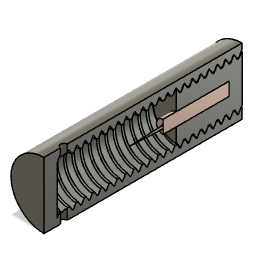
gasChargingBombHolderSchnittbild v2 (Autodesk Fusion 360 design; units mm, degrees)
Autodesk Fusion 360 part; units mm, degrees
sketch "Skizze1" plane through (0, 0, 0) normal (0, 0, 1) x (1, 0, 0)
  circle A0 centre (0, 0) radius 5
  dimension "d1" = 10
  constraint coincident A0.centre origin
  measures "d1" diameter of A0
extrude "Extrusion1" add sketch "Skizze1" along normal blind 10 makes body 1
sketch "Skizze8" plane through (0, 0, 10) normal (0, 0, 1) x (1, 0, 0)
  circle A0 centre (0, 0) radius 5
  circle A1 centre (0, 0) radius 1
  dimension "d45" = 2
  constraint coincident A0.centre A1.centre
  measures "d45" diameter of A1
extrude "Extrusion6" cut sketch "Skizze8" against normal blind 8 contours A1 bodies 1
thread "Gewinde5" "ISO Metric profile 8.0 M8x1.25 6g" major diameter 7.866 minor diameter 6.4455 pitch 1.25 angle 60 modelled right hand crest width 0.1833 on face at (4.9938, -0.2492, 6.6667) crest through (3.933, 0, -0.3125) on bodies 1
sketch "Skizze1 (2)" plane through (0, 0, 0) normal (0, 0, 1) x (1, 0, 0) in component "gasChargingBombLid v4"
  circle A0 centre (0, 0) radius 5
  dimension "d1_1" = 10
  constraint coincident A0.centre origin
  measures "d1_1" diameter of A0
extrude "Extrusion1'" add sketch "Skizze1 (2)" along normal blind 30 separate body makes body 2 in component "gasChargingBombLid v4"
ref_plane "Arbeitsebene1" through (0, 5, 2.1001) normal (0, 1, 0) x (1, 0, 0) in component "gasChargingBombLid v4"
sketch "Skizze3" plane through (0, 5, 2.1001) normal (0, 1, 0) x (1, 0, 0) in component "gasChargingBombLid v4"
  line L0 (-5, 2.1001) -> (5, 2.1001)
  circle A0 centre (0, -0.8999) radius 0.5
  dimension "d16" = 1
  dimension "d17" = 3
  measures "d16" diameter of A0
  measures "d17" distance of L0 A0.centre
sketch "Skizze4" plane through (0, 0, 30) normal (0, 0, 1) x (1, 0, 0) in component "gasChargingBombLid v4"
  circle A0 centre (0, 0) radius 5
  circle A1 centre (0, 0) radius 3.9
  dimension "d12" = 7.8
  constraint concentric A0 A1
  measures "d12" diameter of A1
extrude "Extrusion3" cut sketch "Skizze4" against normal blind 28 contours A1 bodies 2 in component "gasChargingBombLid v4"
extrude "Extrusion4" cut sketch "Skizze3" against normal through all bodies 2 in component "gasChargingBombLid v4"
thread "Gewinde2" "ISO Metric profile 8.0 M8x1.25 6H" major diameter 8.17 minor diameter 6.7795 pitch 1.25 angle 60 modelled right hand crest width 0.343 on face at (3.8806, -0.3883, 11.3333) crest through (3.3898, 0, 29.6875) on bodies 2 in component "gasChargingBombLid v4"
sketch "Skizze9" plane through (0, 0, 2) normal (0, 0, 1) x (1, 0, 0)
  circle A0 centre (0, 0) radius 1
  circle A1 centre (0, 0) radius 1
  constraint coincident A0.centre A1.centre
copy_body "Körper->Berechn1" bodies 1 removing the originals makes body 3 in component "SampleHolder"
sketch "Skizze10" plane through (0, 0, 12) normal (0, 0, 1) x (1, 0, 0)
  circle A0 centre (0, 0) radius 1
  circle A1 centre (0, 0) radius 0.25
  dimension "d51" = 0.5
  constraint coincident A0.centre A1.centre
  measures "d51" diameter of A1
ref_plane "Arbeitsebene2" through (0, 0, 17.5) normal (0, 0, 1) x (1, 0, 0)
sketch "Skizze11" plane through (0, 0, 17.5) normal (0, 0, 1) x (1, 0, 0)
sketch "Skizze1 (3)" plane through (0, 0, 0) normal (0, 1, 0) x (1, 0, 0) in component "Sample v1"
  circle A0 centre (0, 0) radius 1
  circle A1 centre (0, 0) radius 0.25
  dimension "d1_2" = 2
  dimension "d5" = 0.5
  constraint coincident A0.centre A1.centre
  measures "d1_2" diameter of A0
  measures "d5" diameter of A1
ref_plane "Arbeitsebene1" through (0, 5, 0) normal (0, 1, 0) x (0, 0, 1) in component "Sample v1"
sketch "Skizze2" plane through (0, 5, 0) normal (0, 1, 0) x (1, 0, 0) in component "Sample v1"
extrude "Extrusion1''" add sketch "Skizze1 (3)" against normal blind 10 separate body contours A0 | A1 makes body 4 in component "Sample v1"
loft "Erhebung1" add profiles "Skizze1 (3)" section 1 contours A1 section 2 point at (0, 5, 0) separate body makes body 5 in component "Sample v1"
copy_body "Körper->Berechn1'" bodies 4 removing the originals makes body 6 in component "Tube"
copy_body "Körper->Berechn2" bodies 5 removing the originals makes body 7 in component "Sample"
ref_plane "Arbeitsebene3" through (0, 0.0224, 15.0415) normal (1, 0, 0) x (0, 0, -1)
split "Teilen1" by plane through (0, 0, 15) normal (1, 0, 0) bodies 2 makes body 8 at (1.1096, 4.8753, 11) in component "gasChargingBombLid v4"
split "Teilen1'" by plane through (0, 0.0224, 15.0415) normal (1, 0, 0) bodies 3 makes body 9 at (1.693, 1.0752, 0) in component "SampleHolder"
delete_body "Körper entfernen1" bodies 9 in component "SampleHolder"
delete_body "Körper entfernen1'" bodies 8 in component "gasChargingBombLid v4"
split "Teilen1''" by plane through (0, 3.0415, -0.0224) normal (1, 0, 0) bodies 6 makes body 10 at (0.0476, -6.6667, -0.9989) in component "Tube"
split "Teilen1'''" by plane through (0, 3.0415, -0.0224) normal (1, 0, 0) bodies 7 makes body 11 at (0.095, 0.1754, -0.2218) in component "Sample"
delete_body "Körper entfernen1''" bodies 10 in component "Tube"
delete_body "Körper entfernen1'''" bodies 11 in component "Sample"
component "SampleHolder" placed x (1, 0, 0) y (0, 1, 0) z (0, 0, 1) at (0, 0, 0)
component "gasChargingBombLid v4" placed x (1, 0, 0) y (0, -1, 0) z (0, 0, -1) at (0, 0.0224, 30.0415)
component "Sample v1" placed x (1, 0, 0) y (0, 0, 1) z (0, -1, 0) at (0, 0, 12)
component "Tube" placed x (1, 0, 0) y (0, 1, 0) z (0, 0, 1) at (0, 0, 0) in component "Sample v1"
component "Sample" placed x (1, 0, 0) y (0, 1, 0) z (0, 0, 1) at (0, 0, 0) in component "Sample v1"
